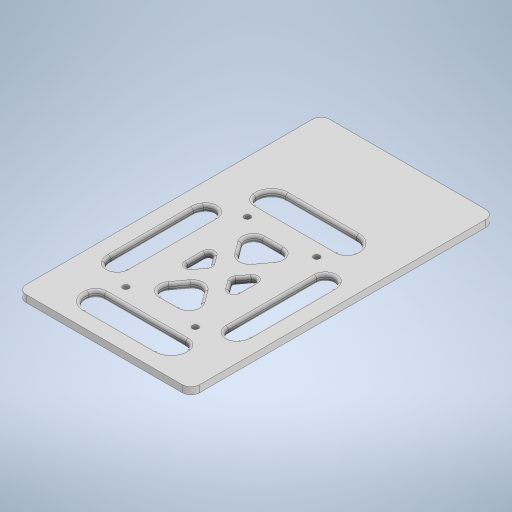
# Autodesk Inventor part: LI0018-NETWORKING SHELF
Saved by Autodesk Inventor 2023 (Build 270158000, 158)
## iProperties
Created: 2023-03-14
Part Number: LI0018-NETWORKING SHELF
Material: Generic
Document SubType Name: Modeling
Designer: Louis
Density: 1 g/cm^3
Appearance: Default
Author: Louis
Autodesk Inventor part; units mm, degrees
ref_plane "YZ Plane" through (0, 0, 0) normal (1, 0, 0) x (0, 1, 0)
ref_plane "XZ Plane" through (0, 0, 0) normal (0, 1, 0) x (-1, 0, 0)
ref_plane "XY Plane" through (0, 0, 0) normal (0, 0, 1) x (1, 0, 0)
sketch "Sketch1" plane through (0, 0, 0) normal (0, 1, 0) x (-1, 0, 0)
  line L0 (50, 67.5) -> (-50, 67.5)
  line L1 (-50, 67.5) -> (-50, -67.5)
  line L2 (-50, -67.5) -> (50, -67.5)
  line L3 (50, -67.5) -> (50, 67.5)
  point P0 (0, 0)
  point P1 (50, 0)
  point P2 (0, 67.5)
  dimension "d0" = 135
  dimension "d1" = 100
  constraints: 8 end point, 2 midpoint, 2 parallel, 1 horizontal, 1 horizontal alignment, 1 perpendicular, 1 vertical alignment
  measures "d0" distance of L2.end L0.start
  measures "d1" distance of L1.end L2.end
extrude "Extrusion1" add sketch "Sketch1" along normal blind 4
sketch "Sketch3" plane through (0, 4, 0) normal (0, 1, 0) x (1, 0, 0)
  line L0 (-25, 40) -> (25, 40)
  line L1 (25, 40) -> (25, -40)
  line L2 (25, -40) -> (-25, -40)
  line L3 (-25, -40) -> (-25, 40)
  line L4 (20, 35) -> (-20, 35)
  line L5 (-20, 35) -> (-20, -35)
  line L6 (-20, -35) -> (20, -35)
  line L7 (20, -35) -> (20, 35)
  point P0 (0, 0)
  point P1 (0, 40)
  point P2 (25, 0)
  point P3 (-20, 35)
  point P4 (20, 35)
  point P5 (-20, -35)
  point P6 (20, -35)
  dimension "d11" = 50
  dimension "d12" = 80
  dimension "d48" = 5
  constraints: 16 end point, 4 coincident, 4 parallel, 2 midpoint, 2 perpendicular, 1 horizontal, 1 horizontal alignment, 1 vertical alignment, 3 other
  measures "d11" distance of L0.start L0.end
  measures "d12" distance of L0.end L1.end
  measures "d48" distance between parallel lines of L0 L4
hole "Hole1" at (-20, 4, -35) at (20, 4, -35) at (-20, 4, 35) at (20, 4, 35) direction (0, -1, 0) diameter 3.4 end through all clearance for "Flat Head Machine Screw" size "M3" standard "Ansi Metric M Profile"
sketch "Sketch4" plane through (0, 4, 0) normal (0, 1, 0) x (1, 0, 0)
  line L0 (-24.5, 39) -> (24.5, 39)
  line L1 (24.5, 39) -> (24.5, -39)
  line L2 (24.5, -39) -> (-24.5, -39)
  line L3 (-24.5, -39) -> (-24.5, 39)
  line L4 (-50, 67.5) -> (50, 67.5)
  line L5 (50, 67.5) -> (50, -67.5)
  line L6 (50, -67.5) -> (-50, -67.5)
  line L7 (-50, -67.5) -> (-50, 67.5)
  line L8 (50, -67.5) -> (50, 67.5) projected
  line L9 (50, 67.5) -> (-50, 67.5) projected
  line L10 (-50, 67.5) -> (-50, -67.5) projected
  line L11 (-50, -67.5) -> (50, -67.5) projected
  line L12 (40, 57.5) -> (-40, 57.5)
  line L13 (-40, 57.5) -> (-40, -57.5)
  line L14 (-40, -57.5) -> (40, -57.5)
  line L15 (40, -57.5) -> (40, 57.5)
  line L16 (29.5, 44) -> (-29.5, 44)
  line L17 (-29.5, 44) -> (-29.5, -44)
  line L18 (-29.5, -44) -> (29.5, -44)
  line L19 (29.5, -44) -> (29.5, 44)
  line L20 (14.5, 29) -> (-14.5, 29)
  line L21 (-14.5, 29) -> (-14.5, -29)
  line L22 (-14.5, -29) -> (14.5, -29)
  line L23 (14.5, -29) -> (14.5, 29)
  line L24 (-50, 67.5) -> (50, -67.5)
  line L25 (50, 67.5) -> (-50, -67.5)
  line L26 (45.9822, 70.4761) -> (-54.0178, -64.5239)
  line L27 (54.0178, 64.5239) -> (-45.9822, -70.4761)
  line L28 (-45.9822, 70.4761) -> (54.0178, -64.5239)
  line L29 (-54.0178, 64.5239) -> (45.9822, -70.4761)
  point P0 (0, 0)
  point P1 (0, 39)
  point P2 (24.5, 0)
  point P3 (50, -62.5)
  point P4 (50, 62.5)
  point P5 (45, 67.5)
  point P6 (-45, 67.5)
  point P7 (-50, 62.5)
  point P8 (-50, -62.5)
  point P9 (-45, -67.5)
  point P10 (45, -67.5)
  point P11 (14.5, -27.9751)
  point P12 (0, -8.4001)
  point P13 (-14.5, -27.9751)
  point P14 (-6.2223, 0)
  point P15 (-14.5, 11.1749)
  point P16 (-14.5, -11.1749)
  point P17 (-14.5, 27.9751)
  point P18 (0, 8.4001)
  point P19 (14.5, 27.9751)
  point P20 (6.2223, 0)
  point P21 (14.5, -11.1749)
  point P22 (14.5, 11.1749)
  point P23 (29.5, -31.4249)
  point P24 (40, -45.5999)
  point P25 (40, 45.5999)
  point P26 (29.5, 31.4249)
  point P27 (36.3703, -57.5)
  point P28 (26.3703, -44)
  point P29 (-26.3703, -44)
  point P30 (-36.3703, -57.5)
  point P31 (-29.5, 31.4249)
  point P32 (-40, 45.5999)
  point P33 (-40, -45.5999)
  point P34 (-29.5, -31.4249)
  point P35 (-36.3703, 57.5)
  point P36 (-26.3703, 44)
  point P37 (26.3703, 44)
  point P38 (36.3703, 57.5)
  point P39 (-29.5, -44.0251)
  point P40 (29.5, -44.0251)
  point P41 (29.5, 44.0251)
  point P42 (-29.5, 44.0251)
  point P43 (-18.9629, 34)
  point P44 (18.9629, 34)
  point P45 (18.9629, -34)
  point P46 (-18.9629, -34)
  dimension "d27" = 10
  dimension "d28" = 5
  dimension "d29" = 10
  dimension "d30" = 5
  dimension "d31" = 5
  dimension "d32" = 5
  dimension "d33" = 5
  dimension "d37" = 49
  dimension "d38" = 78
  constraints: 52 end point, 14 parallel, 5 perpendicular, 4 collinear, 2 horizontal, 2 midpoint, 1 horizontal alignment, 1 vertical alignment, 9 other
  measures "d27" distance between parallel lines of L4 L12
  measures "d28" distance between parallel lines of L0 L16
  measures "d29" distance between parallel lines of L0 L20
  measures "d30" distance between parallel lines of L25 L26
  measures "d31" distance between parallel lines of L25 L27
  measures "d32" distance between parallel lines of L24 L28
  measures "d33" distance between parallel lines of L24 L29
  measures "d37" distance of L0.start L0.end
  measures "d38" distance between parallel lines of L2 L0
extrude "Extrusion3" cut sketch "Sketch4" against normal through all contours L28 L12 L26 L16 | L21 L20 L23 L26 L28 | L17 L26 L13 L29 | L29 L26 L21 | L23 L28 L27 | L27 L15 L28 L19 | L27 L29 L23 L22 L21 | L18 L29 L14 L27
thicken "Thicken1" operation add thickness 40 both sides no extend neighbours no toward (0, 0, -1) faces at (16.6667, 1.3333, -67.5)
fillet "Fillet4" radius 5 4 edges at (-50, 2, -107.5) (50, 2, -107.5) (50, 2, 67.5) (-50, 2, 67.5)
fillet "Fillet5" radius 8 8 edges at (-36.3703, 2, 57.5) (36.3703, 2, 57.5) (40, 2, 45.5999) (40, 2, -45.5999) (36.3703, 2, -57.5) (-36.3703, 2, -57.5) (-40, 2, -45.5999) (-40, 2, 45.5999)
fillet "Fillet6" radius 5 12 edges at (29.5, 2, 31.4249) (29.5, 2, -31.4249) (26.3703, 2, -44) (-26.3703, 2, -44) (-29.5, 2, -31.4249) (-29.5, 2, 31.4249) (26.3703, 2, 44) (-26.3703, 2, 44) (-14.5, 2, 29) (14.5, 2, 29) (14.5, 2, -29) (-14.5, 2, -29)
fillet "Fillet7" radius 2 6 edges at (-14.5, 2, 11.1749) (-6.2223, 2, 0) (-14.5, 2, -11.1749) (14.5, 2, -11.1749) (6.2223, 2, 0) (14.5, 2, 11.1749)
fillet "Fillet8" radius 5 6 edges at (0, 2, 8.4001) (0, 2, -8.4001) (14.5, 2, -27.9751) (-14.5, 2, -27.9751) (-14.5, 2, 27.9751) (14.5, 2, 27.9751)
fillet "Fillet9" radius 1.5 96 edges at (26.6741, 4, 45.1812) (26.5987, 4, 54.664) (0, 4, 57.5) (-26.5987, 4, 54.664) (-26.6741, 4, 45.1812) (0, 4, 44) (-26.6741, 0, 45.1812) (-26.5987, 0, 54.664) (0, 0, 57.5) (26.5987, 0, 54.664) (26.6741, 0, 45.1812) (0, 0, 44) (-39.6594, 4, -26.1349) (-33.0566, 4, -30.271) (-29.5, 4, 0) (-33.0566, 4, 30.271) (-39.6594, 4, 26.1349) (-40, 4, 0) (-39.6594, 0, 26.1349) (-33.0566, 0, 30.271) (-29.5, 0, 0) (-33.0566, 0, -30.271) (-39.6594, 0, -26.1349) (-40, 0, 0) (0, 4, 11.8003) (6.6843, 4, 17.424) (9.7986, 4, 26.2494) (0, 4, 29) (-9.7986, 4, 26.2494) (-6.6843, 4, 17.424) (-9.7986, 0, 26.2494) (0, 0, 29) (9.7986, 0, 26.2494) (6.6843, 0, 17.424) (0, 0, 11.8003) (-6.6843, 0, 17.424) (-13.1268, 4, -7.014) (-8.9985, 4, -3.7479) (-6.7113, 4, 0) (-8.9985, 4, 3.7479) (-13.1268, 4, 7.014) (-14.5, 4, 0) (-13.1268, 0, 7.014) (-8.9985, 0, 3.7479) (-6.7113, 0, 0) (-8.9985, 0, -3.7479) (-13.1268, 0, -7.014) (-14.5, 0, 0) (-9.7986, 4, -26.2494) (0, 4, -29) (9.7986, 4, -26.2494) (6.6843, 4, -17.424) (0, 4, -11.8003) (-6.6843, 4, -17.424) (0, 0, -11.8003) (6.6843, 0, -17.424) (9.7986, 0, -26.2494) (0, 0, -29) (-9.7986, 0, -26.2494) (-6.6843, 0, -17.424) (13.1268, 4, -7.014) (14.5, 4, 0) (13.1268, 4, 7.014) (8.9985, 4, 3.7479) (6.7113, 4, 0) (8.9985, 4, -3.7479) (6.7113, 0, 0) (8.9985, 0, 3.7479) (13.1268, 0, 7.014) (14.5, 0, 0) (13.1268, 0, -7.014) (8.9985, 0, -3.7479) (33.0566, 4, -30.271) (39.6594, 4, -26.1349) (40, 4, 0) (39.6594, 4, 26.1349) (33.0566, 4, 30.271) (29.5, 4, 0) (33.0566, 0, 30.271) (39.6594, 0, 26.1349) (40, 0, 0) (39.6594, 0, -26.1349) (33.0566, 0, -30.271) (29.5, 0, 0) (-26.6741, 4, -45.1812) (-26.5987, 4, -54.664) (0, 4, -57.5) (26.5987, 4, -54.664) (26.6741, 4, -45.1812) (0, 4, -44) (26.6741, 0, -45.1812) (26.5987, 0, -54.664) (0, 0, -57.5) (-26.5987, 0, -54.664) (-26.6741, 0, -45.1812) (0, 0, -44)
body "Solid1"
